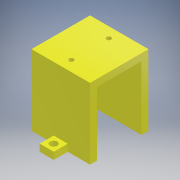
# Autodesk Inventor part: 架子 assembly
Saved by Autodesk Inventor 2017 (Build 210142000, 142)
## iProperties
Created: 2019-12-03
Part Number: 架子 assembly
Material: Generic
Document SubType Name: Modeling
Designer: User
Density: 1 g/cm^3
Appearance: Default
Mass: 6.11436 g
Surface Area: 48.7138 cm^2
Volume: 6.11436 cm^3
Author: User
Autodesk Inventor part; units mm, degrees
ref_plane "YZ Plane" through (0, 0, 0) normal (1, 0, 0) x (0, 1, 0)
ref_plane "XZ Plane" through (0, 0, 0) normal (0, 1, 0) x (-1, 0, 0)
ref_plane "XY Plane" through (0, 0, 0) normal (0, 0, 1) x (1, 0, 0)
sketch "Sketch1" plane through (0, 0, 0) normal (0, 0, 1) x (1, 0, 0)
  line L0 (-12.5, 12.5) -> (12.5, 12.5)
  line L1 (12.5, 12.5) -> (12.5, -12.5)
  line L2 (12.5, -12.5) -> (-12.5, -12.5)
  line L3 (-12.5, -12.5) -> (-12.5, 12.5)
  line L4 (-12.5, 12.5) -> (12.5, -12.5) construction
  line L5 (12.5, 12.5) -> (-12.5, -12.5) construction
  point P0 (0, 0)
  dimension "d0" = 25
  dimension "d1" = 25
  constraints: 12 end point, 2 midpoint, 2 parallel, 1 horizontal, 1 perpendicular
  measures "d0" distance of L1.end L2.end
  measures "d1" distance of L0.end L1.end
extrude "Extrusion1" add sketch "Sketch1" along normal blind 30.25
sketch "Sketch3" plane through (-12.5, -12.5, 0) normal (-1, 0, 0) x (0, 0, 1)
  line L0 (0, 25) -> (0, 0) projected
  line L1 (0, 25) -> (30.25, 25) projected
  line L2 (30.25, 0) -> (30.25, 25) projected
  line L3 (0, 0) -> (30.25, 0) projected
  line L4 (27.25, 3) -> (27.25, 22)
  line L5 (27.25, 22) -> (3, 22)
  line L6 (3, 3) -> (27.25, 3)
  line L7 (3, 3) -> (0, 3)
  line L8 (3, 22) -> (0, 22)
  line L9 (0, 3) -> (0, 22)
  line L10 (0, 0) -> (0, 25) projected
  point P0 (0, 12.5)
  dimension "d16" = 3
  constraints: 12 end point, 2 point on line, 1 collinear, 1 horizontal, 1 other
  measures "d16" distance between parallel lines of L3 L6
sketch "Sketch4" plane through (0, 0, 0) normal (0, 0, -1) x (-1, 0, 0)
  line L0 (3, 18.5) -> (-3, 18.5)
  line L1 (-3, 18.5) -> (-3, 12.5)
  line L2 (-3, 12.5) -> (3, 12.5)
  line L3 (3, 12.5) -> (3, 18.5)
  line L4 (3, 18.5) -> (-3, 12.5) construction
  line L5 (-3, 18.5) -> (3, 12.5) construction
  point P0 (0, 0)
  point P1 (0, 19)
  point P2 (0, 15.5)
  dimension "d19" = 6
  dimension "d20" = 6
  constraints: 12 end point, 2 midpoint, 2 parallel, 1 horizontal, 1 perpendicular
  measures "d19" distance of L2.end L1.end
  measures "d20" distance of L1.end L0.end
extrude "Extrusion3" add sketch "Sketch4" against normal blind 3
mirror "Mirror1" about plane through (0, 0, 0) normal (0, 1, 0) of "Extrusion3"
extrude "Extrusion4" cut sketch "Sketch3" against normal up to next contours L8 L5 L4 L6 L7 L0
sketch "Sketch5" plane through (0, 0, 0) normal (0, 0, -1) x (-1, 0, 0)
  circle A0 centre (0, 15.5) radius 1.55
  point P0 (0, 0)
  dimension "d21" = 3.1
  constraints: 1 centre point
  measures "d21" diameter of A0
extrude "Extrusion5" cut sketch "Sketch5" against normal up to next
mirror "Mirror2" about plane through (0, 0, 0) normal (0, 1, 0) of "Extrusion5"
sketch "Sketch6" plane through (0, 0, 30.25) normal (0, 0, 1) x (1, 0, 0)
  circle A0 centre (0, -8) radius 1
  circle A1 centre (0, 8) radius 1
  point P0 (0, 0)
  dimension "d24" = 2
  dimension "d25" = 2
  constraints: 2 centre point
  measures "d24" diameter of A0
  measures "d25" diameter of A1
extrude "Extrusion6" cut sketch "Sketch6" against normal up to next
body "Solid1"
